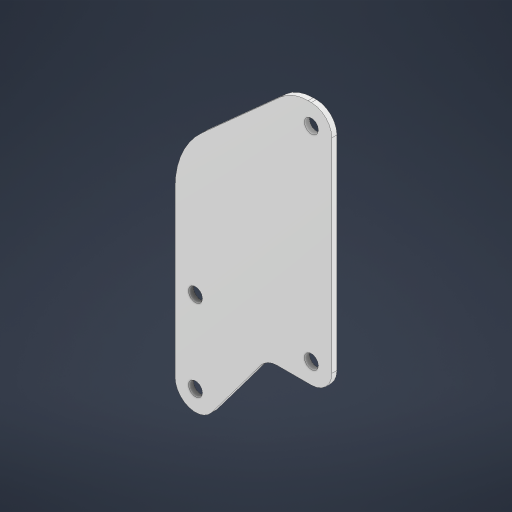
# Autodesk Inventor part: sled
Saved by Autodesk Inventor 2024 (Build 280153000, 153)
## iProperties
Created: 2024-01-16
Part Number: sled
Material: Acetal Resin, White
Document SubType Name: Modeling
Designer: avere
Density: 1.425 g/cm^3
Appearance: Smooth - White
d0: 0.250 in
d1: 0.500 in
Author: avere
Autodesk Inventor part; units mm, degrees
ref_plane "YZ Plane" through (0, 0, 0) normal (1, 0, 0) x (0, 1, 0)
ref_plane "XZ Plane" through (0, 0, 0) normal (0, 1, 0) x (-1, 0, 0)
ref_plane "XY Plane" through (0, 0, 0) normal (0, 0, 1) x (1, 0, 0)
sketch "main" plane through (0, 0, 0) normal (0, 0, 1) x (1, 0, 0)
  arc A0 (15.0953, -24.0958) -> (21.4453, -17.7458) centre (15.0953, -17.7458) ccw
  line L0 (-27.3481, 7.6574) -> (-27.3481, 8.0441)
  circle A1 centre (15.0953, -17.7426) radius 2.1844
  line L1 (15.0953, -24.0958) -> (4.4061, -24.0958)
  arc A2 (4.4061, -24.0958) -> (-0.6731, -26.6347) centre (4.4061, -30.4458) ccw
  circle A3 centre (-20.9981, -17.7426) radius 2.1844
  line L2 (-27.3481, -43.1426) -> (-27.3481, 8.0441)
  line L3 (-15.9189, -46.9536) -> (-0.6731, -26.6347)
  circle A4 centre (-20.9981, -43.1426) radius 2.1844
  arc A5 (-27.3481, -43.1426) -> (-20.9981, -49.4926) centre (-20.9981, -43.1426) ccw
  arc A6 (-27.3481, -43.1426) -> (-15.9189, -46.9536) centre (-20.9981, -43.1426) ccw
  arc A7 (21.4453, 45.7574) -> (15.0953, 52.1074) centre (15.0953, 45.7574) ccw
  arc A8 (-18.881, 26.9766) -> (-27.3481, 8.0441) centre (-1.9481, 8.0441) ccw
  line L4 (21.4453, 45.7574) -> (21.4453, -17.7458)
  line L5 (5.602, 48.8737) -> (-18.881, 26.9766)
  circle A9 centre (15.0953, 45.7574) radius 2.1844
  line L6 (15.0953, 52.1074) -> (14.0684, 52.1074)
  arc A10 (14.0684, 52.1074) -> (5.602, 48.8737) centre (14.0684, 39.4074) ccw
  point P0 (-2.0277, 1.4023)
  point P1 (9.2176, 52.1074)
  dimension "d0" = 6.35
  dimension "d1" = 12.7
  measures "d0" radius of A2
  measures "d1" radius of A10
sketch "Sketch1" plane through (0, 0, 0) normal (0, 0, 1) x (1, 0, 0)
  arc A0 (0, -69.8532) -> (6.35, -63.5032) centre (0, -63.5032) ccw
  line L0 (-42.4434, -38.1) -> (-42.4434, -37.7133)
  circle A1 centre (0, -63.5) radius 2.1844
  line L1 (0, -69.8532) -> (-10.6892, -69.8532)
  arc A2 (-10.6892, -69.8532) -> (-15.7684, -72.3921) centre (-10.6892, -76.2032) ccw
  circle A3 centre (-36.0934, -63.5) radius 2.1844
  line L2 (-42.4434, -88.9) -> (-42.4434, -37.7133)
  line L3 (-31.0142, -92.7111) -> (-15.7684, -72.3921)
  circle A4 centre (-36.0934, -88.9) radius 2.1844
  arc A5 (-42.4434, -88.9) -> (-36.0934, -95.25) centre (-36.0934, -88.9) ccw
  arc A6 (-42.4434, -88.9) -> (-31.0142, -92.7111) centre (-36.0934, -88.9) ccw
  arc A7 (6.35, 0) -> (0, 6.35) centre (0, 0) ccw
  arc A8 (-33.9762, -18.7808) -> (-42.4434, -37.7133) centre (-17.0434, -37.7133) ccw
  line L4 (6.35, 0) -> (6.35, -63.5032)
  line L5 (-9.4933, 3.1162) -> (-33.9762, -18.7808)
  circle A9 centre (0, 0) radius 2.1844
  line L6 (0, 6.35) -> (-1.0269, 6.35)
  arc A10 (-1.0269, 6.35) -> (-9.4933, 3.1162) centre (-1.0269, -6.35) ccw
  point P0 (-42.4434, -38.1)
  constraints: 1 other
extrude "Extrusion1" add sketch "Sketch1" along normal blind 1.5875
body "Solid1"
